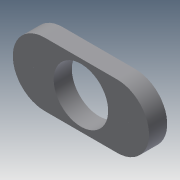
# Autodesk Inventor part: drzak_svetlomet
Saved by Autodesk Inventor 2013 (Build 170138000, 138)
## iProperties
Created: 2014-03-27
Part Number: drzak_svetlomet
Material: Generic
Document SubType Name: Modeling
Designer: idle-rug
Density: 1 g/cm^3
Author: idle-rug
Autodesk Inventor part; units mm, degrees
ref_plane "YZ Plane" through (0, 0, 0) normal (1, 0, 0) x (0, 1, 0)
ref_plane "XZ Plane" through (0, 0, 0) normal (0, 1, 0) x (-1, 0, 0)
ref_plane "XY Plane" through (0, 0, 0) normal (0, 0, 1) x (1, 0, 0)
sketch "Sketch1" plane through (0, 0, 0) normal (0, 1, 0) x (-1, 0, 0)
  line L0 (-20, -17.5) -> (20, -17.5)
  line L1 (20, -17.5) -> (20, 17.5)
  line L2 (20, 17.5) -> (-20, 17.5)
  line L3 (-20, 17.5) -> (-20, -17.5)
  line L4 (-20, -17.5) -> (20, 17.5) construction
  line L5 (20, -17.5) -> (-20, 17.5) construction
  arc A0 (20, -17.5) -> (20, 17.5) centre (20, 0) ccw
  arc A1 (-20, 17.5) -> (-20, -17.5) centre (-20, 0) ccw
  circle A2 centre (0, 0) radius 15
  dimension "d0" = 40
  dimension "d1" = 35
  dimension "d2" = 30
  constraints: 12 end point, 4 point on circle, 4 tangent, 3 centre point, 2 midpoint, 2 parallel, 1 coincident, 1 horizontal, 1 perpendicular
  measures "d0" distance of L2.end L1.end
  measures "d1" distance of L1.end L0.end
  measures "d2" diameter of A2
extrude "Extrusion1" add sketch "Sketch1" along normal blind 10
sketch "Sketch2" plane through (0, 10, 0) normal (0, 1, 0) x (1, 0, 0)
  circle A0 centre (0, 0) radius 15 projected
  arc A1 (20, -17.5) -> (20, 17.5) centre (20, 0) ccw projected
  arc A2 (-20, 17.5) -> (-20, -17.5) centre (-20, 0) ccw projected
  line L0 (-37.5, 0) -> (-15, 0)
  circle A3 centre (0, 0) radius 15 projected
  line L1 (15, 0) -> (37.5, 0)
  circle A4 centre (-26.25, 0) radius 0.1
  circle A5 centre (26.25, 0) radius 0.1
  dimension "d5" = 0.2
  dimension "d6" = 0.2
  constraints: 6 point on circle, 4 end point, 2 centre point, 2 midpoint
  measures "d5" diameter of A4
  measures "d6" diameter of A5
extrude "Extrusion2" cut sketch "Sketch2" against normal blind 10 contours A4 L0 | L0 A4 | A5 L1 | L1 A5
body "Solid1"
